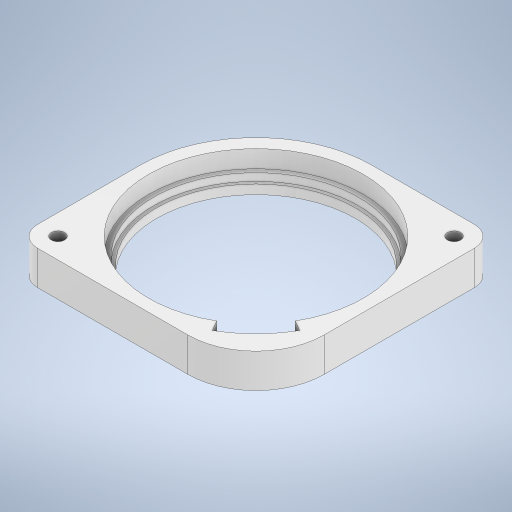
# Autodesk Inventor part: holder
Saved by Autodesk Inventor 2024.3 (Build 283343010, 343A)
## iProperties
Created: 2025-03-09
Part Number: holder
Material: LCP plast
Document SubType Name: Modeling
Designer: hepma_axt67em
Density: 1.626 g/cm^3
Appearance: Hladká – bílá
Author: hepma_axt67em
Autodesk Inventor part; units mm, degrees
ref_plane "YZ Plane" through (0, 0, 0) normal (1, 0, 0) x (0, 1, 0)
ref_plane "XZ Plane" through (0, 0, 0) normal (0, 1, 0) x (-1, 0, 0)
ref_plane "XY Plane" through (0, 0, 0) normal (0, 0, 1) x (1, 0, 0)
sketch "Náčrt1" plane through (0, 0, 0) normal (0, 1, 0) x (-1, 0, 0)
  line L0 (0, -49) -> (0, 49) projected
  line L1 (35, -35) -> (-35, -35)
  line L2 (-35, -35) -> (-35, 35)
  line L3 (-35, 35) -> (35, 35)
  line L4 (35, 35) -> (35, -35)
  line L5 (-49, 0) -> (49, 0) projected
  dimension "d9" = 70
  dimension "d10" = 70
  constraints: 8 end point, 2 parallel, 1 horizontal, 1 perpendicular, 2 other
  measures "d9" distance of L1.end L2.end
  measures "d10" distance of L1.start L1.end
extrude "Vysunutí1" add sketch "Náčrt1" along normal blind 10
fillet "Zaoblení1" radius 6 2 edges at (35, 5, -35) (-35, 5, 35)
fillet "Zaoblení2" radius 34 1 edges at (-35, 5, -35)
sketch "Náčrt2" plane through (0, 10, 0) normal (0, 1, 0) x (1, 0, 0)
  line L0 (0, 49) -> (0, -49) projected
  line L1 (49, 0) -> (-49, 0) projected
  point P0 (0, 0)
  point P1 (0, 0)
  constraints: 1 coincident
hole "Díra1" at (0, 10, 0) direction (0, -1, 0) diameter 60.1 depth 7.3 counterbore diameter 62.9 counterbore depth 5.1
sketch "Náčrt3" plane through (0, 2.7, 0) normal (0, 1, 0) x (1, 0, 0)
  line L0 (0, 49) -> (0, -49) projected
  line L1 (49, 0) -> (-49, 0) projected
  point P0 (0, 0)
  point P1 (0, 0)
  constraints: 1 coincident
hole "Díra2" at (0, 2.7, 0) direction (0, -1, 0) diameter 58.2 end through all
sketch "Náčrt4" plane through (0, 10, 0) normal (0, 1, 0) x (1, 0, 0)
  arc A0 (-35, -29) -> (-29, -35) centre (-29, -29) ccw projected
  arc A1 (35, 29) -> (29, 35) centre (29, 29) ccw projected
  point P0 (0, 0)
  constraints: 2 coincident
hole "Díra3" at (-29, 10, 29) at (29, 10, -29) direction (0, -1, 0) diameter 3.9 end through all
sketch "Náčrt5" plane through (0, 10, 0) normal (0, 1, 0) x (1, 0, 0)
  arc A0 (17.5, -30.3109) -> (30.3109, -17.5) centre (0, 0) ccw
  line L0 (0, 49) -> (0, -49) projected
  line L1 (49, 0) -> (-49, 0) projected
  line L2 (0, 0) -> (17.5, -30.3109)
  line L3 (30.3109, -17.5) -> (0, 0)
  dimension "d35" = 35
  dimension "d36" = 30
  dimension "d37" = 30
  constraints: 4 end point, 2 point on circle, 1 centre point, 1 coincident
  measures "d35" radius of A0
  measures "d36" angle of L1 L3
  measures "d37" angle of L0 L2
extrude "Vysunutí2" cut sketch "Náčrt5" against normal up to surface (10 mm away)
fillet "Zaoblení4" radius 20 1 edges at (35, 5, 35)
